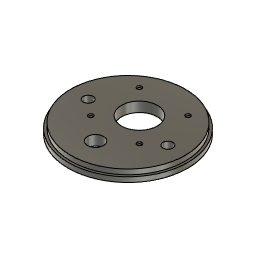
BulkPlate_Stepper_Mount_SubScale v1 (Autodesk Fusion 360 design; units mm, degrees)
Autodesk Fusion 360 part; units mm, degrees
sketch "Sketch1" plane through (0, 0, 0) normal (0, 0, 1) x (1, 0, 0)
  circle A0 centre (0, 0) radius 38.0746
  dimension "d1" = 76.1492
  constraint coincident A0.centre origin
  measures "d1" diameter of A0
extrude "Extrude1" add sketch "Sketch1" along normal blind 3.175
sketch "Sketch2" plane through (0, 0, 3.175) normal (0, 0, 1) x (-1, 0, 0)
  circle A0 centre (0, 0) radius 38.0746
  circle A1 centre (0, 0) radius 36.5125
  dimension "d4" = 73.025
  constraint coincident A0.centre A1.centre
  measures "d4" diameter of A1
extrude "Extrude2" add sketch "Sketch2" along normal blind 3.175 contours A1
sketch "Sketch3" plane through (0, 0, 6.35) normal (0, 0, 1) x (-1, 0, 0)
  circle A0 centre (0, 0) radius 36.5125
  circle A1 centre (25.4, 0) radius 3.175
  circle A2 centre (-25.4, 0) radius 3.175
  circle A3 centre (0, -7.2644) radius 11.43
  circle A4 centre (0, 20.6756) radius 5.08
  circle A5 centre (0, 0) radius 38.0746
  dimension "d7" = 6.35
  dimension "d8" = 6.35
  dimension "d9" = 50.8
  dimension "d10" = 25.4
  dimension "d11" = 10.16
  dimension "d12" = 20.6756
  dimension "d13" = 22.86
  dimension "d14" = 27.94
  measures "d7" diameter of A1
  measures "d8" diameter of A2
  measures "d9" distance of A1.centre A2.centre
  measures "d10" distance of A0.centre A2.centre
  measures "d11" diameter of A4
  measures "d12" distance of A4.centre A0.centre
  measures "d13" diameter of A3
  measures "d14" distance of A3.centre A4.centre
extrude "Extrude3" cut sketch "Sketch3" against normal blind 22.86 contours A1 | A2 | A3 | A4
sketch "Sketch4" plane through (0, 0, 6.35) normal (0, 0, 1) x (-1, 0, 0)
  circle A0 centre (-25.4, 0) radius 3.175
  circle A1 centre (0, 20.6756) radius 5.08
  circle A2 centre (0, -7.2644) radius 11.43
  circle A3 centre (25.4, 0) radius 3.175
  circle A4 centre (0, 0) radius 36.5125
  circle A5 centre (15.494, -22.7584) radius 1.4986
  circle A6 centre (15.494, 8.2296) radius 1.4986
  circle A7 centre (-15.494, 8.2296) radius 1.4986
  circle A8 centre (-15.494, -22.7584) radius 1.4986
  dimension "d17" = 2.9972
  dimension "d18" = 30.988
  dimension "d19" = 15.494
  dimension "d20" = 15.494
  dimension "d21" = 30.988
  constraint horizontal A5.centre A8.centre
  constraint vertical A5.centre A6.centre
  constraint horizontal A6.centre A7.centre
  constraint vertical A7.centre A8.centre
  constraint equal A5 A8
  constraint equal A7 A8
  constraint equal A6 A7
  measures "d17" diameter of A5
  measures "d18" distance of A5.centre A6.centre
  measures "d19" vertical distance of A2.centre A6.centre
  measures "d20" horizontal distance of A2.centre A6.centre
  measures "d21" distance of A5.centre A8.centre
extrude "Extrude4" cut sketch "Sketch4" against normal blind 1.016 contours A5 | A6 | A7 | A8
